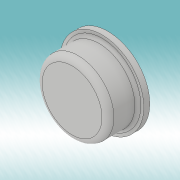
# Autodesk Inventor part: Foot
Saved by Autodesk Inventor 2019 (Build 230136000, 136)
## iProperties
Created: 2019-01-31
Part Number: Foot
Material: Generic
Document SubType Name: Modeling
Designer: USUARIO
Density: 1 g/cm^3
Appearance: Default
Author: USUARIO
Autodesk Inventor part; units mm, degrees
ref_plane "YZ Plane" through (0, 0, 0) normal (1, 0, 0) x (0, 1, 0)
ref_plane "XZ Plane" through (0, 0, 0) normal (0, 1, 0) x (-1, 0, 0)
ref_plane "XY Plane" through (0, 0, 0) normal (0, 0, 1) x (1, 0, 0)
sketch "Sketch1" plane through (0, 0, 0) normal (0, 0, 1) x (1, 0, 0)
  line L0 (0, 0) -> (16, 0)
  line L1 (16, 0) -> (16, 16)
  line L2 (16, 16) -> (0, 16)
  line L3 (0, 16) -> (0, 0)
  circle A0 centre (8, 8) radius 7
  dimension "d0" = 16
  dimension "d1" = 8
  dimension "d2" = 8
  dimension "d3" = 14
  constraints: 8 end point, 2 parallel, 2 perpendicular, 1 centre point, 1 horizontal
  measures "d0" distance of L2.end L1.end
  measures "d1" distance from line of L2 A0.centre
  measures "d2" distance from line of L1 A0.centre
  measures "d3" diameter of A0
extrude "Extrusion2" add sketch "Sketch1" along normal blind 1 contours A0
sketch "Sketch3" plane through (8, 8, 1) normal (0, 0, 1) x (1, 0, 0)
  circle A0 centre (0, 0) radius 6
  circle A1 centre (0, 0) radius 7 projected
  point P0 (-8, -8)
  dimension "d10" = 12
  constraints: 1 centre point, 1 concentric
  measures "d10" diameter of A0
extrude "Extrusion3" add sketch "Sketch3" along normal blind 5 contours A0
fillet "Fillet1" radius 1 1 edges at (2, 8, 6)
fillet "Fillet1" radius 0.5 1 edges at (2, 8, 1)
body "Solid2"
